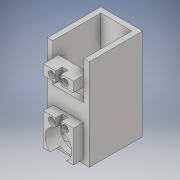
# Autodesk Inventor part: BasePlateBottom
Saved by Autodesk Inventor 2018 (Build 220112000, 112)
## iProperties
Created: 2018-06-26
Part Number: BasePlateBottom
Material: Generic
Document SubType Name: Modeling
Designer: brend
Density: 1 g/cm^3
Appearance: Default
Author: brend
Autodesk Inventor part; units mm, degrees
ref_plane "YZ Plane" through (0, 0, 0) normal (1, 0, 0) x (0, 1, 0)
ref_plane "XZ Plane" through (0, 0, 0) normal (0, 1, 0) x (-1, 0, 0)
ref_plane "XY Plane" through (0, 0, 0) normal (0, 0, 1) x (1, 0, 0)
sketch "Sketch1" plane through (0, 0, 0) normal (0, 0, 1) x (1, 0, 0)
  line L0 (0, 0) -> (19.939, 0)
  line L1 (19.939, 0) -> (19.939, 25.4)
  line L2 (19.939, 25.4) -> (0, 25.4)
  line L3 (0, 25.4) -> (0, 0)
  dimension "d0" = 19.939
  dimension "d1" = 25.4
  constraints: 8 end point, 2 parallel, 1 horizontal, 1 perpendicular
  measures "d0" distance of L2.end L1.end
  measures "d1" distance of L1.end L0.end
extrude "Extrusion1" add sketch "Sketch1" along normal blind 25.4
shell "Shell1" thickness 2.54 removed faces 1 at (13.2927, 25.4, 8.4667)
sketch "Sketch2" plane through (0, 0, 25.4) normal (0, 0, 1) x (1, 0, 0)
  line L0 (15.367, 1.905) -> (4.572, 1.905)
  line L1 (4.572, 1.905) -> (4.572, 17.145)
  line L2 (4.572, 17.145) -> (15.367, 17.145)
  line L3 (15.367, 17.145) -> (15.367, 1.905)
  line L4 (15.367, 1.905) -> (4.572, 17.145) construction
  line L5 (4.572, 1.905) -> (15.367, 17.145) construction
  line L6 (0, 25.4) -> (0, 0) projected
  line L7 (0, 0) -> (19.939, 0) projected
  circle A0 centre (9.9695, 6.985) radius 3.175
  circle A1 centre (6.7945, 14.9098) radius 1.5875
  circle A2 centre (13.1318, 14.9098) radius 1.5875
  line L8 (19.939, 0) -> (19.939, 25.4) projected
  point P0 (9.9695, 9.525)
  dimension "d5" = 9.9695
  dimension "d6" = 9.525
  dimension "d7" = 15.24
  dimension "d8" = 10.795
  dimension "d9" = 6.35
  dimension "d10" = 5.08
  dimension "d11" = 3.175
  dimension "d12" = 7.9248
  dimension "d13" = 3.175
  dimension "d15" = 6.7945
  dimension "d16" = 6.8072
  dimension "d24" = 6.985
  constraints: 12 end point, 3 centre point, 2 midpoint, 2 parallel, 1 horizontal, 1 perpendicular
  measures "d5" distance from line of L6 point (9.97, 9.525)
  measures "d6" distance from line of L7 point (9.97, 9.525)
  measures "d7" distance between parallel lines of L2 L0
  measures "d8" distance between parallel lines of L1 L3
  measures "d9" diameter of A0
  measures "d10" distance from line of L0 A0.centre
  measures "d11" diameter of A1
  measures "d12" vertical distance of A1.centre A0.centre
  measures "d13" diameter of A2
  measures "d15" distance from line of L6 A1.centre
  measures "d16" distance from line of L8 A2.centre
  measures "d24" distance from line of L7 A0.centre
hole "Hole1" at (13.1318, 14.9098, 25.4) at (6.7945, 14.9098, 25.4) direction (0, 0, -1) diameter 3.175 depth 7.62 tip angle 118
sketch "Sketch3" plane through (0, 0, 25.4) normal (0, 0, 1) x (1, 0, 0)
  circle A0 centre (9.9695, 6.985) radius 6.35
  line L0 (0, 0) -> (19.939, 0) projected
  line L1 (19.939, 0) -> (19.939, 25.4) projected
  dimension "d25" = 12.7
  dimension "d26" = 6.985
  dimension "d27" = 9.9695
  constraints: 1 centre point
  measures "d25" diameter of A0
  measures "d26" distance from line of L0 A0.centre
  measures "d27" distance from line of L1 A0.centre
hole "Hole2" at (9.9695, 6.985, 25.4) direction (0, 0, -1) diameter 12.7 depth 2.54 tip angle 118
sketch "Sketch4" plane through (0, 0, 25.4) normal (0, 0, 1) x (1, 0, 0)
  line L0 (17.1577, 1.905) -> (2.8067, 1.905)
  line L1 (2.8067, 1.905) -> (2.8067, 17.145)
  line L2 (2.8067, 17.145) -> (17.1577, 17.145)
  line L3 (17.1577, 17.145) -> (17.1577, 1.905)
  line L4 (17.1577, 1.905) -> (2.8067, 17.145) construction
  line L5 (2.8067, 1.905) -> (17.1577, 17.145) construction
  line L6 (0, 0) -> (19.939, 0) projected
  line L7 (0, 25.4) -> (0, 0) projected
  circle A0 centre (13.1318, 14.9352) radius 1.5875
  circle A1 centre (6.7945, 14.9352) radius 1.5875
  line L8 (19.939, 0) -> (19.939, 25.4) projected
  circle A2 centre (9.9695, 6.985) radius 6.35
  point P0 (9.9822, 9.525)
  dimension "d35" = 9.525
  dimension "d36" = 14.351
  dimension "d38" = 9.9822
  dimension "d39" = 6.8072
  dimension "d40" = 6.7945
  dimension "d41" = 12.7
  dimension "d42" = 9.9695
  dimension "d43" = 5.08
  dimension "d44" = 7.9502
  dimension "d45" = 7.9502
  dimension "d56" = 6.3373
  dimension "d66" = 1.905
  dimension "d75" = 2.8067
  dimension "d76" = 2.7813
  constraints: 12 end point, 3 centre point, 2 midpoint, 2 parallel, 1 horizontal, 1 perpendicular
  measures "d35" distance from line of L6 point (9.982, 9.525)
  measures "d36" distance from line of L3 L0.end
  measures "d38" distance from line of L7 point (9.982, 9.525)
  measures "d39" distance from line of L8 A0.centre
  measures "d40" distance from line of L7 A1.centre
  measures "d41" diameter of A2
  measures "d42" distance from line of L7 A2.centre
  measures "d43" distance from line of L0 A2.centre
  measures "d44" vertical distance of A2.centre A0.centre
  measures "d45" vertical distance of A2.centre A1.centre
  measures "d56" distance of A0.centre A1.centre
  measures "d66" distance between parallel lines of L6 L0
  measures "d75" distance between parallel lines of L7 L1
  measures "d76" distance between parallel lines of L8 L3
sketch "Sketch5" plane through (0, 0, 25.4) normal (0, 0, 1) x (1, 0, 0)
  point P0 (0, 0)
extrude "Extrusion2" add sketch "Sketch4" along normal blind 4.7625 contours L0 A2 L1 L2 L3
sketch "Sketch6" plane through (0, 0, 30.1625) normal (0, 0, 1) x (1, 0, 0)
  line L0 (17.1577, 1.905) -> (2.8067, 1.905) projected
  line L1 (8.6487, 1.905) -> (11.3157, 1.905)
  line L2 (11.3157, 1.905) -> (11.3157, 40.005)
  line L3 (11.3157, 40.005) -> (8.6487, 40.005)
  line L4 (8.6487, 40.005) -> (8.6487, 1.905)
  line L5 (17.1577, 1.905) -> (17.1577, 17.145) projected
  point P0 (0, 0)
  dimension "d48" = 2.667
  dimension "d49" = 5.842
  dimension "d71" = 38.1
  constraints: 8 end point, 2 parallel, 1 horizontal, 1 perpendicular, 1 point on line
  measures "d48" distance of L3.end L2.end
  measures "d49" distance between parallel lines of L5 L2
  measures "d71" distance between parallel lines of L3 L0
extrude "Extrusion3" cut sketch "Sketch6" against normal blind 3.175
sketch "Sketch9" plane through (2.54, 2.54, 2.54) normal (0, 0, 1) x (1, 0, 0)
  line L0 (1.8542, 12.7) -> (6.9342, 12.7)
  line L1 (6.9342, 12.7) -> (6.9342, 7.9375)
  line L2 (6.9342, 7.9375) -> (1.8542, 7.9375)
  line L3 (1.8542, 7.9375) -> (1.8542, 12.7)
  line L4 (7.9375, 12.7) -> (14.2875, 12.7)
  line L5 (14.2875, 12.7) -> (14.2875, 7.9375)
  line L6 (14.2875, 7.9375) -> (7.9375, 7.9375)
  line L7 (7.9375, 7.9375) -> (7.9375, 12.7)
  line L8 (0, 22.86) -> (14.859, 22.86) projected
  line L9 (0, 22.86) -> (0, 0) projected
  point P0 (-2.54, -2.54)
  dimension "d97" = 10.16
  dimension "d98" = 5.08
  dimension "d100" = 1.8542
  dimension "d101" = 4.7625
  constraints: 16 end point, 4 parallel, 2 horizontal, 2 perpendicular
  measures "d97" distance between parallel lines of L8 L0
  measures "d98" distance between parallel lines of L3 L1
  measures "d100" distance between parallel lines of L9 L3
  measures "d101" distance between parallel lines of L2 L0
extrude "Extrusion5" add sketch "Sketch9" along normal blind 5.08 contours L0 L1 L2 L3
sketch "Sketch10" plane through (2.54, 2.54, 2.54) normal (0, 0, 1) x (1, 0, 0)
  line L0 (7.9375, 7.9375) -> (13.0175, 7.9375)
  line L1 (13.0175, 7.9375) -> (13.0175, 12.7)
  line L2 (13.0175, 12.7) -> (7.9375, 12.7)
  line L3 (7.9375, 12.7) -> (7.9375, 7.9375)
  line L4 (0, 22.86) -> (14.859, 22.86) projected
  line L5 (1.8542, 12.7) -> (6.9342, 12.7) projected
  point P0 (-2.54, -2.54)
  dimension "d94" = 5.08
  dimension "d95" = 10.16
  dimension "d96" = 10.16
  dimension "d99" = 1.8415
  dimension "d102" = 4.7625
  constraints: 8 end point, 2 parallel, 1 horizontal, 1 perpendicular
  measures "d94" distance between parallel lines of L3 L1
  measures "d95" distance between parallel lines of L2 L4
  measures "d96" distance between parallel lines of L4 L5
  measures "d99" distance from line of L4.end L1
  measures "d102" distance between parallel lines of L0 L2
extrude "Extrusion6" add sketch "Sketch10" along normal blind 5.08
sketch "Sketch11" plane through (0, 0, 0) normal (0, 0, -1) x (-1, 0, 0)
  circle A0 centre (-13.1445, 12.7) radius 1.5875
  circle A1 centre (-6.7945, 12.7) radius 1.5875
  line L0 (0, 25.4) -> (0, 0) projected
  line L1 (-19.939, 0) -> (-19.939, 25.4) projected
  line L2 (0, 0) -> (-19.939, 0) projected
  dimension "d81" = 6.7945
  dimension "d91" = 12.7
  dimension "d92" = 12.7
  dimension "d93" = 6.35
  constraints: 2 centre point
  measures "d81" distance from line of L0 A1.centre
  measures "d91" distance from line of L2 A1.centre
  measures "d92" distance from line of L2 A0.centre
  measures "d93" distance of A1.centre A0.centre
hole "Hole4" at (13.1445, 12.7, 0) at (6.7945, 12.7, 0) direction (0, 0, 1) diameter 3.175 depth 15.24 tip angle 118
sketch "Sketch12" plane through (0, 25.4, 0) normal (0, 1, 0) x (1, 0, 0)
  line L0 (0, 0) -> (0, -25.4) projected
  line L1 (19.939, 0) -> (19.939, -25.4) projected
  line L2 (0, 0) -> (19.939, 0)
  line L3 (19.939, 0) -> (19.939, -25.4)
  line L4 (19.939, -25.4) -> (0, -25.4)
  line L5 (0, -25.4) -> (0, 0)
  constraints: 8 end point, 2 parallel, 1 horizontal, 1 perpendicular
extrude "Extrusion7" add sketch "Sketch12" along normal blind 18.1429
sketch "Sketch13" plane through (0, 43.5429, 0) normal (0, 1, 0) x (1, 0, 0)
  line L0 (2.54, -2.54) -> (17.399, -2.54)
  line L1 (17.399, -2.54) -> (17.399, -25.4)
  line L2 (17.399, -25.4) -> (2.54, -25.4)
  line L3 (2.54, -25.4) -> (2.54, -2.54)
  line L4 (19.939, 0) -> (0, 0) projected
  line L5 (0, 0) -> (0, -25.4) projected
  line L6 (19.939, -25.4) -> (19.939, 0) projected
  dimension "d105" = 2.54
  dimension "d106" = 2.54
  dimension "d107" = 25.4
  dimension "d110" = 2.54
  constraints: 8 end point, 2 parallel, 1 horizontal, 1 perpendicular
  measures "d105" distance between parallel lines of L4 L0
  measures "d106" distance between parallel lines of L5 L3
  measures "d107" distance between parallel lines of L4 L2
  measures "d110" distance between parallel lines of L6 L1
extrude "Extrusion8" cut sketch "Sketch13" against normal blind 18.1429
sketch "Sketch14" plane through (0, 0, 25.4) normal (0, 0, 1) x (1, 0, 0)
  line L0 (2.8067, 36.5125) -> (17.1577, 36.5125)
  line L1 (17.1577, 36.5125) -> (17.1577, 31.75)
  line L2 (17.1577, 31.75) -> (2.8067, 31.75)
  line L3 (2.8067, 31.75) -> (2.8067, 36.5125)
  line L4 (0, 0) -> (0, 43.5429) projected
  line L5 (19.939, 0) -> (19.939, 43.5429) projected
  line L6 (2.8067, 17.145) -> (2.8067, 1.905) projected
  line L7 (17.1577, 1.905) -> (17.1577, 17.145) projected
  dimension "d134" = 0
  dimension "d135" = 0
  constraints: 8 end point, 2 parallel, 1 horizontal, 1 perpendicular
  measures "d134" distance between parallel lines of L6 L3
  measures "d135" distance between parallel lines of L7 L1
extrude "Extrusion9" add sketch "Sketch14" along normal blind 4.7625 and the other way blind 2.54
sketch "Sketch15" plane through (0, 0, 30.1625) normal (0, 0, 1) x (1, 0, 0)
  line L0 (2.8067, 31.75) -> (17.1577, 31.75) projected
  line L1 (8.6487, 31.75) -> (11.3157, 31.75)
  line L2 (11.3157, 31.75) -> (11.3157, 36.5125)
  line L3 (11.3157, 36.5125) -> (8.6487, 36.5125)
  line L4 (8.6487, 36.5125) -> (8.6487, 31.75)
  line L5 (2.8067, 36.5125) -> (2.8067, 31.75) projected
  line L6 (17.1577, 31.75) -> (17.1577, 36.5125) projected
  line L7 (17.1577, 36.5125) -> (2.8067, 36.5125) projected
  line L8 (19.939, 0) -> (19.939, 43.5429) projected
  line L9 (17.399, 43.5429) -> (17.399, 25.4) projected
  line L10 (17.1577, 1.905) -> (17.1577, 17.145) projected
  point P0 (0, 0)
  point P1 (17.399, 31.75)
  dimension "d119" = 0
  dimension "d130" = 2.667
  dimension "d133" = 5.842
  constraints: 8 end point, 2 parallel, 1 horizontal, 1 perpendicular, 1 point on line
  measures "d119" distance between parallel lines of L7 L3
  measures "d130" distance between parallel lines of L2 L4
  measures "d133" distance between parallel lines of L10 L2
extrude "Extrusion10" cut sketch "Sketch15" against normal blind 3.175 contours L4 L3 L2 L0
sketch "Sketch16" plane through (0, 0, 30.1625) normal (0, 0, 1) x (1, 0, 0)
  circle A0 centre (6.8072, 34.0179) radius 1.5875
  circle A1 centre (13.1318, 34.0179) radius 1.5875
  line L0 (0, 0) -> (0, 43.5429) projected
  line L1 (19.939, 0) -> (19.939, 43.5429) projected
  line L2 (2.54, 43.5429) -> (17.399, 43.5429) projected
  dimension "d122" = 3.175
  dimension "d123" = 3.175
  dimension "d124" = 6.8072
  dimension "d125" = 6.8072
  dimension "d126" = 9.525
  dimension "d127" = 9.525
  constraints: 2 centre point
  measures "d122" diameter of A0
  measures "d123" diameter of A1
  measures "d124" distance from line of L0 A0.centre
  measures "d125" distance from line of L1 A1.centre
  measures "d126" distance from line of L2 A0.centre
  measures "d127" distance from line of L2 A1.centre
extrude "Extrusion11" cut sketch "Sketch16" against normal blind 12.7
sketch "Sketch17" plane through (0, 0, 25.4) normal (0, 0, 1) x (1, 0, 0)
  line L0 (17.1577, 36.5125) -> (17.1577, 31.75) projected
  line L1 (19.939, 0) -> (19.939, 43.5429) projected
  line L2 (17.1577, 31.75) -> (19.939, 31.75)
  line L3 (19.939, 31.75) -> (19.939, 36.5125)
  line L4 (19.939, 36.5125) -> (17.1577, 36.5125)
  line L5 (17.1577, 36.5125) -> (17.1577, 31.75)
  line L6 (2.8067, 31.75) -> (2.8067, 36.5125) projected
  line L7 (0, 0) -> (0, 43.5429) projected
  line L8 (2.8067, 31.75) -> (0, 31.75)
  line L9 (0, 31.75) -> (0, 36.5125)
  line L10 (0, 36.5125) -> (2.8067, 36.5125)
  line L11 (2.8067, 36.5125) -> (2.8067, 31.75)
  constraints: 16 end point, 4 parallel, 3 point on line, 2 horizontal, 2 perpendicular
extrude "Extrusion12" add sketch "Sketch17" against normal blind 2.54
equation "\"d125\" = d124"
equation "\"d127\" = d126"
body "Solid1"
